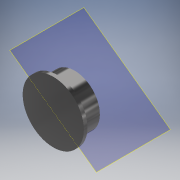
# Autodesk Inventor part: lid
Saved by Autodesk Inventor 2018 (Build 220112000, 112)
## iProperties
Created: 2017-10-26
Part Number: lid
Material: Stainless Steel
Document SubType Name: Modeling
Designer: kurtis
Density: 8 g/cm^3
Appearance: Semi-Polished
Author: kurtis
Autodesk Inventor part; units mm, degrees
ref_plane "YZ Plane" through (0, 0, 0) normal (1, 0, 0) x (0, 1, 0)
ref_plane "XZ Plane" through (0, 0, 0) normal (0, 1, 0) x (-1, 0, 0)
ref_plane "XY Plane" through (0, 0, 0) normal (0, 0, 1) x (1, 0, 0)
ref_plane "Work Plane1" through (56.2325, -3.9241, -54.643) normal (0.9843, -0.1766, 0) x (0.1766, 0.9843, 0)
sketch "Sketch1" plane through (56.2325, -3.9241, -54.643) normal (0.9843, -0.1766, 0) x (0.1766, 0.9843, 0)
  line L0 (8.8813, -28.7707) -> (8.8813, -26.2307) construction
  line L1 (8.8813, -26.2307) -> (11.7241, -26.2307) construction
  line L2 (11.7241, -26.2307) -> (11.7241, -28.7707) construction
  line L3 (11.7241, -28.7707) -> (8.8813, -28.7707) construction
  line L4 (4.5958, -26.2307) -> (4.5958, -28.7707) construction
  line L5 (4.5958, -28.7707) -> (-5.2462, -28.7707) construction
  line L6 (-5.2462, -28.7707) -> (-5.2462, -26.2307) construction
  line L7 (-5.2462, -26.2307) -> (4.5958, -26.2307) construction
  line L8 (19.4818, -26.2307) -> (19.4818, -28.7707) construction
  line L9 (19.4818, -28.7707) -> (16.7961, -28.7707) construction
  line L10 (16.7961, -28.7707) -> (16.7961, -26.2307) construction
  line L11 (16.7961, -26.2307) -> (19.4818, -26.2307) construction
  spline S0 degree 2 poles (40.7352, 49.563) (36.4181, 6.3217) (32.911, -28.7707) knots 0 0 0 7.872352 7.872352 7.872352 weights 1 1.005429 1 construction
  line L12 (32.911, -28.7707) -> (24.0815, -28.7707) construction
  line L13 (24.0815, -28.7707) -> (24.0815, -26.2307) construction
  line L14 (24.0815, -26.2307) -> (30.6156, -26.2307) construction
  spline S1 degree 2 poles (30.6156, -26.2307) (33.9974, 7.5872) (38.19, 49.563) knots 0 0 0 7.617126 7.617126 7.617126 weights 1 1.005811 1 construction
  line L15 (38.19, 49.563) -> (38.4437, 52.103) construction
  line L16 (38.4437, 52.103) -> (48.6252, 52.103) construction
  line L17 (48.6252, 52.103) -> (48.6252, 43.213) construction
  line L18 (48.6252, 43.213) -> (46.0815, 43.213) construction
  line L19 (46.0815, 43.213) -> (46.0815, 49.563) construction
  line L20 (46.0815, 49.563) -> (40.7352, 49.563) construction
  spline S2 degree 2 poles (-34.4769, -28.7707) (-37.984, 6.3217) (-42.3012, 49.563) knots 0 0 0 7.872352 7.872352 7.872352 weights 1 1.005429 1 construction
  line L21 (-42.3012, 49.563) -> (-47.6475, 49.563) construction
  line L22 (-47.6475, 49.563) -> (-47.6475, 43.213) construction
  line L23 (-47.6475, 43.213) -> (-50.1911, 43.213) construction
  line L24 (-50.1911, 43.213) -> (-50.1911, 52.103) construction
  line L25 (-50.1911, 52.103) -> (-40.0096, 52.103) construction
  line L26 (-40.0096, 52.103) -> (-39.7559, 49.563) construction
  spline S3 degree 2 poles (-39.7559, 49.563) (-35.5633, 7.5872) (-32.1815, -26.2307) knots 0 0 0 7.617126 7.617126 7.617126 weights 1 1.005811 1 construction
  line L27 (-32.1815, -26.2307) -> (-8.6835, -26.2307) construction
  line L28 (-8.6835, -26.2307) -> (-8.6835, -28.7707) construction
  line L29 (-8.6835, -28.7707) -> (-34.4769, -28.7707) construction
  line L30 (43.5344, 52.103) -> (43.5344, 57.183)
  line L31 (43.5344, 52.103) -> (40.9944, 52.103)
  line L32 (40.9944, 52.103) -> (40.9944, 54.643)
  line L33 (40.9944, 54.643) -> (35.9144, 54.643)
  line L34 (35.9144, 54.643) -> (35.9144, 26.7834)
  line L35 (35.9144, 26.7834) -> (33.3744, 26.7834)
  line L36 (33.3744, 26.7834) -> (33.3744, 54.643)
  line L37 (33.3744, 54.643) -> (0, 54.643)
  line L38 (0, 57.183) -> (43.5344, 57.183)
  line L39 (0, 57.183) -> (0, 54.643)
  point P0 (-6.0665, 54.643)
  dimension "d1" = 5.08
  dimension "d4" = 2.54
  dimension "d5" = 2.54
  dimension "d6" = 5.08
  dimension "d7" = 2.54
  dimension "d8" = 2.54
  dimension "d9" = 48.6252
  constraints: 78 end point, 17 horizontal, 14 vertical, 3 perpendicular, 2 point on line, 1 midpoint, 1 parallel, 52 other
  measures "d1" distance of L30.start L30.end
  measures "d4" distance of L30.start L31.end
  measures "d5" distance of L31.end L32.end
  measures "d6" distance of L32.end L33.end
  measures "d7" distance of L34.end L35.end
  measures "d8" distance of L38.start L37.end
  measures "d9" distance from line of L16.end L39
revolve "Revolution1" add sketch "Sketch1" angle 360 about axis through (56.2325, -3.9241, 2.54) along (0, 0, -1)
body "Solid1"
